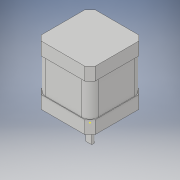
# Autodesk Inventor part: nema17_84Ncm
Saved by Autodesk Inventor 2018 (Build 220112000, 112)
## iProperties
Created: 2020-03-14
Part Number: nema17_84Ncm
Material: Generic
Document SubType Name: Modeling
Designer: natha
Density: 1 g/cm^3
Appearance: Default
Author: natha
Autodesk Inventor part; units mm, degrees
ref_plane "YZ Plane" through (0, 0, 0) normal (1, 0, 0) x (0, 1, 0)
ref_plane "XZ Plane" through (0, 0, 0) normal (0, 1, 0) x (-1, 0, 0)
ref_plane "XY Plane" through (0, 0, 0) normal (0, 0, 1) x (1, 0, 0)
sketch "Sketch1" plane through (0, 0, 0) normal (0, 1, 0) x (-1, 0, 0)
  line L0 (0, 0) -> (42, 0)
  line L1 (42, 0) -> (42, -42)
  line L2 (42, -42) -> (0, -42)
  line L3 (0, -42) -> (0, 0)
  dimension "d0" = 42
  dimension "d1" = 42
  constraints: 8 end point, 2 parallel, 1 horizontal, 1 perpendicular
  measures "d0" distance of L1.end L2.end
  measures "d1" distance of L0.end L1.end
extrude "Extrusion1" add sketch "Sketch1" along normal blind 10
chamfer "Chamfer1" distance 4 angle 45 4 edges at (0, 5, 0) (0, 5, -42) (-42, 5, -42) (-42, 5, 0)
sketch "Sketch2" plane through (0, 10, 0) normal (0, 1, 0) x (1, 0, 0)
  point P0 (0, 0)
sketch "Sketch3" plane through (0, 10, 0) normal (0, 1, 0) x (1, 0, 0)
  line L0 (-0.5, 0.5) -> (-41.5, 0.5)
  line L1 (-41.5, 0.5) -> (-41.5, 41.5)
  line L2 (-41.5, 41.5) -> (-0.5, 41.5)
  line L3 (-0.5, 41.5) -> (-0.5, 0.5)
  line L4 (-0.5, 0.5) -> (-41.5, 41.5) construction
  line L5 (-41.5, 0.5) -> (-0.5, 41.5) construction
  point P0 (0, 0)
  point P1 (-21, 21)
  dimension "d7" = 41
  dimension "d8" = 41
  constraints: 12 end point, 2 midpoint, 2 parallel, 1 horizontal, 1 perpendicular
  measures "d7" distance of L1.end L2.end
  measures "d8" distance of L0.end L1.end
extrude "Extrusion2" add sketch "Sketch3" along normal blind 26
fillet "Fillet1" radius 6.35 4 edges at (-41.5, 23, -41.5) (-0.5, 23, -41.5) (-41.5, 23, -0.5) (-0.5, 23, -0.5)
sketch "Sketch4" plane through (0, 36, 0) normal (0, 1, 0) x (1, 0, 0)
  line L0 (0, 0) -> (-42, 0)
  line L1 (-42, 0) -> (-42, 42)
  line L2 (-42, 42) -> (0, 42)
  line L3 (0, 42) -> (0, 0)
  dimension "d12" = 42
  dimension "d13" = 42
  constraints: 8 end point, 2 parallel, 1 horizontal, 1 perpendicular
  measures "d12" distance of L1.end L2.end
  measures "d13" distance of L0.end L1.end
extrude "Extrusion3" add sketch "Sketch4" along normal blind 10
chamfer "Chamfer2" distance 4 angle 45 4 edges at (-42, 41, -42) (-42, 41, 0) (0, 41, -42) (0, 41, 0)
sketch "Sketch5" plane through (0, 0, 0) normal (0, -1, 0) x (1, 0, 0)
  circle A0 centre (-21, -21) radius 11
  point P0 (0, 0)
  dimension "d19" = 22
  constraints: 1 centre point
  measures "d19" diameter of A0
extrude "Extrusion4" add sketch "Sketch5" along normal blind 2
sketch "Sketch6" plane through (-21, -2, -21) normal (0, -1, 0) x (1, 0, 0)
  circle A0 centre (0, 0) radius 2.5
  point P0 (21, 21)
  dimension "d22" = 5
  constraints: 1 centre point
  measures "d22" diameter of A0
extrude "Extrusion5" add sketch "Sketch6" along normal blind 22
sketch "Sketch7" plane through (0, 0, 0) normal (0, -1, 0) x (1, 0, 0)
  circle A0 centre (-37, -5) radius 1.5
  circle A1 centre (-5, -5) radius 1.5
  circle A2 centre (-5, -37) radius 1.5
  circle A3 centre (-37, -37) radius 1.5
  point P0 (0, 0)
  dimension "d25" = 3
  dimension "d26" = 3
  dimension "d27" = 3
  dimension "d28" = 3
  constraints: 4 centre point
  measures "d25" diameter of A0
  measures "d26" diameter of A1
  measures "d27" diameter of A2
  measures "d28" diameter of A3
extrude "Extrusion6" cut sketch "Sketch7" against normal blind 3
sketch "Sketch8" plane through (-21, -24, -21) normal (0, -1, 0) x (1, 0, 0)
  circle A0 centre (0, 0) radius 2.5 projected
  arc A1 (-2.2228, 1.1442) -> (2.2228, 1.1442) centre (0, 0) ccw
  line L0 (-2.2228, 1.1442) -> (2.2228, 1.1442)
  point P0 (21, 21)
  constraints: 4 point on circle, 2 end point, 1 centre point, 1 horizontal
extrude "Extrusion7" cut sketch "Sketch8" against normal blind 22 contours L0 A0 picked at (0.2976, 1.8759)
body "Solid1"
